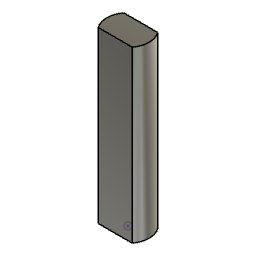
NEW extended shaft 1 (Autodesk Fusion 360 design; units mm, degrees)
Autodesk Fusion 360 part; units mm, degrees
sketch "Sketch1" plane through (0, 0, 0) normal (0, 0, 1) x (1, 0, 0)
  line L0 (0, 1.5) -> (-2, 1.5)
  line L1 (0, 1.5) -> (2, 1.5)
  arc A0 (-2, 1.5) -> (-2, -1.5) centre (0, 0) ccw
  arc A1 (2, -1.5) -> (2, 1.5) centre (0, 0) ccw
  circle A2 centre (0, 0) radius 3.5
  line L2 (-2, -1.5) -> (2, -1.5)
  dimension "d2" = 5
  dimension "d3" = 1.5
  dimension "d5" = 7
  constraint coincident A0.centre A1.centre
  constraint coincident A1.start A0
  constraint concentric A0 A1
  constraint horizontal L2
  measures "d2" diameter of A0
  measures "d3" distance of A0.centre L0.start
  measures "d5" diameter of A2
extrude "Extrude1" add sketch "Sketch1" along normal blind 20 contours L0 L1 A0 A1 L2
sketch "Sketch2" plane through (0, 0, 0) normal (0, 0, 1) x (1, 0, 0)
